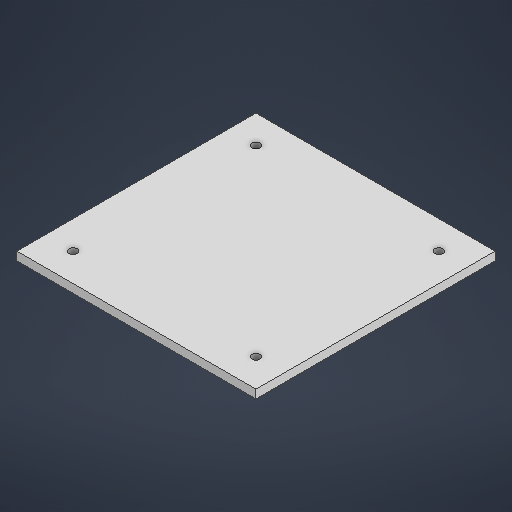
# Autodesk Inventor part: topLid
Saved by Autodesk Inventor 2026.2 (Build 302298000, 298)
## iProperties
Created: 2026-09-25
Part Number: topLid
Material: Generic
Document SubType Name: Modeling
Designer: Brian Wang
Density: 1 g/cm^3
Appearance: Default
Author: Brian Wang
Autodesk Inventor part; units mm, degrees
ref_plane "YZ Plane" through (0, 0, 0) normal (1, 0, 0) x (0, 1, 0)
ref_plane "XZ Plane" through (0, 0, 0) normal (0, 1, 0) x (-1, 0, 0)
ref_plane "XY Plane" through (0, 0, 0) normal (0, 0, 1) x (1, 0, 0)
sketch "Sketch1" plane through (0, 0, 0) normal (0, 1, 0) x (-1, 0, 0)
  line L0 (9.5438, 13.8424) -> (-75.4562, 13.8424)
  line L1 (-75.4562, 13.8424) -> (-75.4562, -71.1576)
  line L2 (-75.4562, -71.1576) -> (9.5438, -71.1576)
  line L3 (9.5438, -71.1576) -> (9.5438, 13.8424)
  circle A0 centre (-0.4562, 3.8424) radius 1.5
  circle A1 centre (-0.4562, -61.1576) radius 1.5
  circle A2 centre (-65.4562, -61.1576) radius 1.5
  circle A3 centre (-65.4562, 3.8424) radius 1.5
  point P0 (0, 0)
  dimension "d0" = 85
  dimension "d1" = 85
  dimension "d2" = 3
  dimension "d3" = 3
  dimension "d4" = 3
  dimension "d5" = 3
  dimension "d6" = 10
  dimension "d7" = 10
  dimension "d8" = 10
  dimension "d9" = 10
  dimension "d10" = 10
  dimension "d11" = 10
  dimension "d12" = 10
  dimension "d13" = 10
  dimension "d14" = 65
  constraints: 8 end point, 4 centre point, 2 horizontal alignment, 2 parallel, 2 vertical alignment, 1 horizontal, 1 perpendicular
  measures "d0" distance of L2.end L1.end
  measures "d1" distance of L1.end L0.end
  measures "d2" diameter of A0
  measures "d3" diameter of A1
  measures "d4" diameter of A2
  measures "d5" diameter of A3
  measures "d6" distance from line of L3 A0.centre
  measures "d7" distance from line of L0 A0.centre
  measures "d8" distance from line of L2 A1.centre
  measures "d9" distance from line of L3 A1.centre
  measures "d10" distance from line of L2 A2.centre
  measures "d11" distance from line of L1 A2.centre
  measures "d12" distance from line of L0 A3.centre
  measures "d13" distance from line of L1 A3.centre
  measures "d14" distance of A3.centre A0.centre
extrude "Extrusion1" add sketch "Sketch1" along normal blind 3
body "Solid1"
